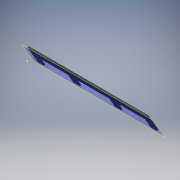
# Autodesk Inventor part: 칼팁
Saved by Autodesk Inventor 2017 (Build 210142000, 142)
## iProperties
Part Number: 칼팁
Material: 철, 주조
Document SubType Name: Modeling
Designer: Minos
Mass: 49.9429 g
Surface Area: 84.0875 cm^2
Volume: 6.98502 cm^3
Density: 7.15 g/cm^3
Appearance: 철 회색
Author: Minos
Autodesk Inventor part; units mm, degrees
note: some values were not read from the file. Chosen so that the rebuilt part matches the saved one: sketch regions of "돌출1".
ref_plane "YZ Plane" through (0, 0, 0) normal (1, 0, 0) x (0, 1, 0)
ref_plane "XZ Plane" through (0, 0, 0) normal (0, 1, 0) x (-1, 0, 0)
ref_plane "작업 평면1" through (126.678, -21.6572, 32.6995) normal (0, 0.8660254, 0.5) x (1, 0, 0)
sketch "스케치1" plane through (126.678, -21.6572, 32.6995) normal (0, 0.8660254, 0.5) x (1, 0, 0)
  circle A0 centre (89.9, 9) radius 1.5 projected
  circle A1 centre (-89.9, -1) radius 1.5 projected
  circle A2 centre (-89.9, 9) radius 1.5 projected
  circle A3 centre (89.9, -1) radius 1.5 projected
  circle A4 centre (32.9, 9) radius 1.5 projected
  circle A5 centre (-32.9, -1) radius 1.5 projected
  circle A6 centre (-32.9, 9) radius 1.5 projected
  circle A7 centre (32.9, -1) radius 1.5 projected
  line L0 (95, -17) -> (95, 17) projected
  line L1 (8, 17) -> (95, 17) projected
  line L2 (8, 17) -> (8, 10) projected
  arc A8 (6, 8) -> (8, 10) centre (6, 10) ccw projected
  line L3 (6, 8) -> (-6, 8) projected
  arc A9 (-8, 10) -> (-6, 8) centre (-6, 10) ccw projected
  line L4 (-8, 10) -> (-8, 17) projected
  line L5 (-95, 17) -> (-8, 17) projected
  line L6 (-95, 17) -> (-95, -17) projected
  line L7 (95, -17) -> (-95, -17) projected
  line L8 (95, 13) -> (95, -20)
  line L9 (95, -20) -> (-95, -20)
  line L10 (-95, -20) -> (-95, 13)
  line L11 (-95, 13) -> (-84.8, 13)
  line L12 (-84.8, 13) -> (-84.8, -5)
  line L13 (-84.8, -5) -> (-95, -5)
  line L14 (-95, -5) -> (-95, 13)
  line L15 (-38, 13) -> (-27.8, 13)
  line L16 (-27.8, 13) -> (-27.8, -5)
  line L17 (-27.8, -5) -> (-38, -5)
  line L18 (-38, -5) -> (-38, 13)
  line L19 (27.8, 13) -> (38, 13)
  line L20 (38, 13) -> (38, -5)
  line L21 (38, -5) -> (27.8, -5)
  line L22 (27.8, -5) -> (27.8, 13)
  line L23 (95, 13) -> (84.8, 13)
  line L24 (84.8, 13) -> (84.8, -5)
  line L25 (84.8, -5) -> (95, -5)
  line L26 (95, -5) -> (95, 13)
  line L27 (-84.8, -5) -> (84.8, -5)
  line L28 (84.8, 13) -> (95, 13)
  line L29 (27.8, 13) -> (38, 13)
  line L30 (-95, 13) -> (-84.8, 13)
  line L31 (-38, 13) -> (-27.8, 13)
  point P0 (-126.678, 39.1472)
  dimension "d1" = 190
  dimension "d2" = 33
  dimension "d5" = 10.2
  dimension "d6" = 18
  dimension "d7" = 10.2
  dimension "d8" = 18
  dimension "d9" = 10.2
  dimension "d10" = 18
  dimension "d11" = 5.1
  dimension "d12" = 18
  dimension "d13" = 10.2
  dimension "d14" = 5.1
  constraints: 48 end point, 13 parallel, 8 horizontal, 8 perpendicular, 2 point on line
  measures "d1" distance of L8.end L9.end
  measures "d2" distance of L8.start L8.end
  measures "d5" distance of L12.end L13.end
  measures "d6" distance of L11.end L12.end
  measures "d7" distance of L25.end L24.end
  measures "d8" distance of L24.end L23.end
  measures "d9" distance of L20.end L21.end
  measures "d10" distance of L21.end L19.start
  measures "d11" distance from line of L22 A4.centre
  measures "d12" distance of L17.end L15.start
  measures "d13" distance of L16.end L17.end
  measures "d14" distance from line of L16 A5.centre
extrude "돌출1" add sketch "스케치1" along normal blind 2 contours L7 L6 L13 L27 L17 L21 L25 L0 | L8 L9 L10 L7 | L25 L24 L23 L0 | L6 L11 L12 L13 | L21 L22 L19 L20 | L18 L15 L16 L17
sketch "스케치2" plane through (126.678, -19.9251, 33.6995) normal (0, 0.8660254, 0.5) x (1, 0, 0)
  circle A0 centre (32.9, 9) radius 1.5 projected
  circle A1 centre (32.9, -1) radius 1.5 projected
  circle A2 centre (-89.9, 9) radius 1.5 projected
  circle A3 centre (-89.9, -1) radius 1.5 projected
  circle A4 centre (89.9, 9) radius 1.5 projected
  circle A5 centre (89.9, -1) radius 1.5 projected
  circle A6 centre (-32.9, 9) radius 1.5 projected
  circle A7 centre (-32.9, -1) radius 1.5 projected
  line L0 (-38, 13) -> (-38, -5) projected
  line L1 (-38, -5) -> (-84.8, -5) projected
  line L2 (-84.8, -5) -> (-84.8, 13) projected
  line L3 (-84.8, 13) -> (-95, 13) projected
  line L4 (-95, 13) -> (-95, -20) projected
  line L5 (-95, -20) -> (95, -20) projected
  line L6 (95, -20) -> (95, 13) projected
  line L7 (95, 13) -> (84.8, 13) projected
  line L8 (84.8, 13) -> (84.8, -5) projected
  line L9 (84.8, -5) -> (38, -5) projected
  line L10 (38, -5) -> (38, 13) projected
  line L11 (38, 13) -> (27.8, 13) projected
  line L12 (27.8, 13) -> (27.8, -5) projected
  line L13 (27.8, -5) -> (-27.8, -5) projected
  line L14 (-27.8, -5) -> (-27.8, 13) projected
  line L15 (-27.8, 13) -> (-38, 13) projected
  line L16 (-95, -20) -> (95, -20) projected
  line L17 (-86, -20) -> (-86, -12)
  line L18 (-86, -12) -> (-70, -12)
  line L19 (-70, -12) -> (-50, -12)
  line L20 (-50, -12) -> (-30, -12)
  line L21 (-30, -12) -> (-10, -12)
  line L22 (-10, -12) -> (10, -12)
  line L23 (10, -12) -> (30, -12)
  line L24 (30, -12) -> (50, -12)
  line L25 (50, -12) -> (70, -12)
  line L26 (70, -12) -> (86, -12)
  circle A8 centre (-86, -12) radius 1.5
  circle A9 centre (-70, -12) radius 1.5
  circle A10 centre (-50, -12) radius 1.5
  circle A11 centre (-30, -12) radius 1.5
  circle A12 centre (-10, -12) radius 1.5
  circle A13 centre (10, -12) radius 1.5
  circle A14 centre (30, -12) radius 1.5
  circle A15 centre (50, -12) radius 1.5
  circle A16 centre (70, -12) radius 1.5
  circle A17 centre (86, -12) radius 1.5
  point P0 (-126.678, 39.1472)
  dimension "d17" = 8
  dimension "d18" = 16
  dimension "d19" = 20
  dimension "d20" = 20
  dimension "d21" = 20
  dimension "d22" = 20
  dimension "d23" = 20
  dimension "d24" = 20
  dimension "d25" = 20
  dimension "d26" = 16
  dimension "d27" = 9
  dimension "d28" = 3
  dimension "d29" = 3
  dimension "d30" = 3
  dimension "d31" = 3
  dimension "d32" = 3
  dimension "d33" = 3
  dimension "d34" = 3
  dimension "d35" = 3
  dimension "d36" = 3
  dimension "d38" = 3
  constraints: 20 end point, 10 centre point, 9 point on line, 2 perpendicular, 1 coincident
  measures "d17" distance of L17.start L17.end
  measures "d18" distance of L17.end L18.end
  measures "d19" distance of L18.end L19.end
  measures "d20" distance of L19.end L20.end
  measures "d21" distance of L20.end L21.end
  measures "d22" distance of L21.end L22.end
  measures "d23" distance of L22.end L23.end
  measures "d24" distance of L23.end L24.end
  measures "d25" distance of L24.end L25.end
  measures "d26" distance of L25.end L26.end
  measures "d27" distance between parallel lines of L17 L4
  measures "d28" diameter of A8
  measures "d29" diameter of A9
  measures "d30" diameter of A10
  measures "d31" diameter of A11
  measures "d32" diameter of A12
  measures "d33" diameter of A13
  measures "d34" diameter of A14
  measures "d35" diameter of A15
  measures "d36" diameter of A16
  measures "d38" diameter of A17
extrude "돌출2" cut sketch "스케치2" against normal blind 1 contours A8 L18 L17 | L17 L18 A8 | A9 L19 L18 | L18 L19 A9 | A10 L20 L19 | L19 L20 A10 | A11 L21 L20 | L20 L21 A11 | A12 L22 L21 | L21 L22 A12 | A13 L23 L22 | L22 L23 A13 | A14 L24 L23 | L23 L24 A14 | A15 L25 L24 | L24 L25 A15 | A16 L26 L25 | L25 L26 A16 | A17
